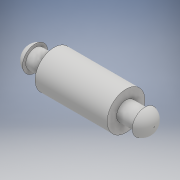
# Autodesk Inventor part: Reverse Gear LInk Rod
Saved by Autodesk Inventor 2017 (Build 210142000, 142)
## iProperties
Created: 2018-11-17
Part Number: Reverse Gear LInk Rod
Material: Generic
Document SubType Name: Modeling
Designer: Arman Grewal
Density: 1 g/cm^3
Appearance: Default
Author: Arman Grewal
Autodesk Inventor part; units mm, degrees
ref_plane "XZ Plane" through (0, 0, 0) normal (0, 1, 0) x (-1, 0, 0)
ref_plane "XY Plane" through (0, 0, 0) normal (0, 0, 1) x (1, 0, 0)
sketch "Sketch1" plane through (0, 0, 0) normal (1, 0, 0) x (0, 1, 0)
  circle A0 centre (0, 0) radius 3
  dimension "d0" = 6
  constraints: 1 centre point, 1 coincident
  measures "d0" diameter of A0
extrude "Extrusion1" add sketch "Sketch1" along normal blind 11.5
sketch "Sketch2" plane through (11.5, 0, 0) normal (1, 0, 0) x (0, 0, -1)
  circle A0 centre (0, 0) radius 1.5
  dimension "d3" = 3
  constraints: 1 centre point, 1 coincident
  measures "d3" diameter of A0
extrude "Extrusion2" add sketch "Sketch2" along normal blind 3
sketch "Sketch3" plane through (0, 0, 0) normal (0, 1, 0) x (-1, 0, 0)
  line L0 (-14.5, 1.5) -> (-14.5, -1.5) projected
  line L1 (-14.5, 0) -> (-14.5, 2)
  line L2 (-14.5, 0) -> (-14.5, -2)
  line L3 (-14.5, -2) -> (-16, -2)
  line L4 (-14.5, 2) -> (-16, 2)
  line L5 (-16, 2) -> (-16, -2)
  point P0 (0, 0)
  dimension "d6" = 2
  dimension "d7" = 2
  dimension "d8" = 1.5
  constraints: 10 end point, 2 perpendicular, 2 vertical, 1 horizontal, 1 midpoint
  measures "d6" distance of L1.start L1.end
  measures "d7" distance of L1.start L2.end
  measures "d8" distance of L2.end L3.end
extrude "Extrusion3" add sketch "Sketch3" along normal mid plane 4
fillet "Fillet1" radius 2 4 edges at (15.25, 2, -2) (15.25, 2, 2) (15.25, -2, 2) (15.25, -2, -2)
fillet "Fillet2" radius 2 8 edges at (16, 0, -2) (16, 1.4142, -1.4142) (16, -1.4142, -1.4142) (16, 2, 0) (16, -2, 0) (16, 1.4142, 1.4142) (16, -1.4142, 1.4142) (16, 0, 2)
ref_plane "Work Plane1" through (5.75, 0, 0) normal (1, 0, 0) x (0, 1, 0)
mirror "Mirror1" about plane through (5.75, 0, 0) normal (1, 0, 0) of "Extrusion2"
sketch "Sketch4" plane through (0, 0, 0) normal (0, 1, 0) x (-1, 0, 0)
  line L0 (3, 1.5) -> (3, -1.5) projected
  line L1 (3, 0) -> (3, 2)
  line L2 (3, 2) -> (3, -2)
  line L3 (3, -2) -> (4.5, -2)
  line L4 (4.5, -2) -> (4.5, 2)
  line L5 (4.5, 2) -> (3, 2)
  point P0 (0, 0)
  dimension "d14" = 2
  dimension "d15" = 4
  dimension "d16" = 1.5
  constraints: 10 end point, 2 perpendicular, 1 collinear, 1 horizontal, 1 midpoint, 1 point on line
  measures "d14" distance of L1.start L1.end
  measures "d15" distance of L1.end L2.end
  measures "d16" distance of L2.end L3.end
extrude "Extrusion4" add sketch "Sketch4" along normal mid plane 4
fillet "Fillet3" radius 2 4 edges at (-3.75, 2, 2) (-3.75, 2, -2) (-3.75, -2, 2) (-3.75, -2, -2)
fillet "Fillet4" radius 2 8 edges at (-4.5, 2, 0) (-4.5, 1.4142, 1.4142) (-4.5, 1.4142, -1.4142) (-4.5, 0, 2) (-4.5, 0, -2) (-4.5, -1.4142, 1.4142) (-4.5, -1.4142, -1.4142) (-4.5, -2, 0)
body "Solid1"
